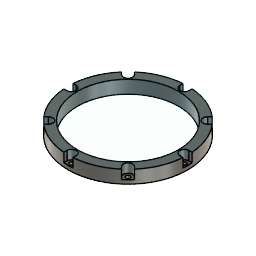
CycloidalDriveV1Assembly (Autodesk Fusion 360 archive; units mm, degrees)
design "CoperchioOutput2.0"
part number: 2026-04-16-14-40-12-138
Autodesk Fusion 360 part; units mm, degrees
sketch "Sketch1" plane through (0, 0, 0) normal (0, 0, 1) x (1, 0, 0)
  circle A0 centre (0, 0) radius 46
  circle A1 centre (0, 0) radius 38.925
  dimension "d1" = 92
  dimension "d2" = 77.85
  constraint coincident A0.centre A1.centre
  constraint concentric A0 A1
  measures "d1" diameter of A0
  measures "d2" diameter of A1
extrude "Extrude1" add sketch "Sketch1" along normal blind 10
sketch "Sketch2" plane through (0, 0, 10) normal (0, 0, 1) x (-1, 0, 0)
  circle A0 centre (0, 0) radius 38.925
  circle A1 centre (0, 0) radius 46
  circle A2 centre (0, -43.375) radius 1.65
  dimension "d5" = 3.3
  dimension "d6" = 43.375
  measures "d5" diameter of A2
  measures "d6" distance of A0.centre A2.centre
extrude "Extrude2" cut sketch "Sketch2" against normal blind 10 contours A2
sketch "Sketch3" plane through (0, 0, 10) normal (0, 0, 1) x (-1, 0, 0)
  circle A0 centre (0, -43.375) radius 1.65
  circle A1 centre (0, 0) radius 38.925
  circle A2 centre (0, 0) radius 46
pattern_circular "C-Pattern1" count 8 over 360 about axis through (0, 0, 1.75) along (0, 0, 1) of "Extrude2"
sketch "Sketch4" plane through (0, 0, 10) normal (0, 0, 1) x (-1, 0, 0)
  circle A0 centre (0, -43.375) radius 1.65
  line L0 (3.5, -43.375) -> (3.5, -46)
  line L1 (-3.5, -43.375) -> (-3.5, -46)
  arc A1 (3.5, -43.375) -> (-3.5, -43.375) centre (0, -43.375) ccw
  circle A2 centre (0, 0) radius 46
  dimension "d11" = 7
  constraint concentric A0 A1
  constraint tangent L0 A1
  constraint vertical L0
  constraint tangent L1 A1
  constraint vertical L1
  measures "d11" diameter of A1
extrude "Extrude3" cut sketch "Sketch4" against normal blind 7 contours L0 L1 A1 A2 picked at (-2.8289, -44.4442)
pattern_circular "C-Pattern2" count 8 over 360 about axis through (0, 0, 1.75) along (0, 0, 1) of "Extrude3"

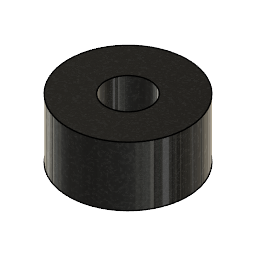
design "Cuscinetto 3x8x4"
part number: 2026-04-13-20-27-40-353
Autodesk Fusion 360 part; units mm, degrees
sketch "Sketch1" plane through (0, 0, 0) normal (0, 0, 1) x (1, 0, 0)
  circle A0 centre (0, 0) radius 1.5
  circle A1 centre (0, 0) radius 4
  dimension "d1" = 3
  dimension "d2" = 8
  constraint coincident A0.centre A1.centre
  constraint concentric A0 A1
  measures "d1" diameter of A0
  measures "d2" diameter of A1
extrude "Extrude1" add sketch "Sketch1" along normal blind 4

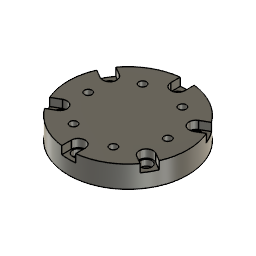
design "Output8mm2.0"
part number: 2026-04-23-17-57-34-450
Autodesk Fusion 360 part; units mm, degrees
sketch "Sketch1" plane through (0, 0, 0) normal (0, 0, 1) x (1, 0, 0)
  circle A0 centre (0, 0) radius 30
  dimension "d1" = 60
  constraint coincident A0.centre origin
  measures "d1" diameter of A0
extrude "Extrude1" add sketch "Sketch1" along normal blind 7
sketch "Sketch2" plane through (0, 0, 7) normal (0, 0, 1) x (-1, 0, 0)
  circle A0 centre (0, 0) radius 30
  line L0 (0, 0) -> (0, -25) construction
  circle A1 centre (0, -25) radius 2.825
  dimension "d4" = 5.65
  constraint coincident A0.centre L0.start
  constraint vertical L0
  constraint coincident L0.end A1.centre
  measures "d4" diameter of A1
extrude "Extrude2" cut sketch "Sketch2" against normal blind 3 contours A1
sketch "Sketch3" plane through (0, 0, 4) normal (0, 0, 1) x (-1, 0, 0)
  circle A0 centre (0, -25) radius 2.825
  circle A1 centre (0, -25) radius 1.675
  dimension "d7" = 3.35
  constraint concentric A0 A1
  measures "d7" diameter of A1
extrude "Extrude3" cut sketch "Sketch3" against normal blind 4 contours A1
pattern_circular "C-Pattern1" count 6 over 360 about axis through (0, 0, 1.75) along (0, 0, 1) of "Extrude2", "Extrude3"
sketch "Sketch5" plane through (0, 0, 7) normal (0, 0, 1) x (-1, 0, 0)
  circle A0 centre (0, 0) radius 30
  circle A1 centre (0, -25) radius 2.825
  circle A2 centre (21.6506, -12.5) radius 2.825
  circle A3 centre (21.6506, 12.5) radius 2.825
  circle A4 centre (0, 25) radius 2.825
  circle A5 centre (-21.6506, 12.5) radius 2.825
  circle A6 centre (-21.6506, -12.5) radius 2.825
  line L0 (-3.5, 25) -> (-3.5, 29.7951)
  line L1 (3.5, 25) -> (3.5, 29.7951)
  line L2 (0, 25) -> (0, 30) construction
  arc A7 (-3.5, 25) -> (3.5, 25) centre (0, 25) ccw
  circle A8 centre (0, 0) radius 30
  line L3 (-23.4006, 9.4689) -> (-27.5533, 11.8665)
  arc A9 (-23.4006, 9.4689) -> (-19.9006, 15.5311) centre (-21.6506, 12.5) ccw
  line L4 (-19.9006, 15.5311) -> (-24.0533, 17.9287)
  line L5 (-19.9006, -15.5311) -> (-24.0533, -17.9287)
  arc A10 (-19.9006, -15.5311) -> (-23.4006, -9.4689) centre (-21.6506, -12.5) ccw
  line L6 (-23.4006, -9.4689) -> (-27.5533, -11.8665)
  line L7 (3.5, -25) -> (3.5, -29.7951)
  arc A11 (3.5, -25) -> (-3.5, -25) centre (0, -25) ccw
  line L8 (-3.5, -25) -> (-3.5, -29.7951)
  line L9 (23.4006, -9.4689) -> (27.5533, -11.8665)
  arc A12 (23.4006, -9.4689) -> (19.9006, -15.5311) centre (21.6506, -12.5) ccw
  line L10 (19.9006, -15.5311) -> (24.0533, -17.9287)
  line L11 (19.9006, 15.5311) -> (24.0533, 17.9287)
  arc A13 (19.9006, 15.5311) -> (23.4006, 9.4689) centre (21.6506, 12.5) ccw
  line L12 (23.4006, 9.4689) -> (27.5533, 11.8665)
  dimension "d16" = 7
  dimension "d18" = 360
  constraint concentric A4 A7
  constraint coincident A0 L0.end
  constraint vertical L0
  constraint tangent L0 A7
  constraint coincident A0 L1.end
  constraint tangent L1 A7
  constraint coincident A4.centre L2.start
  constraint coincident A0 L2.end
  constraint vertical L2
  measures "d16" diameter of A7
extrude "Extrude5" add sketch "Sketch5" along normal blind 4 contours A0 L0 L1 A7 A8 L3 A9 L4 L5 A10 L6 L7 A11 L8 L9 A12 L10 L11 A13 L12
sketch "Sketch6" plane through (0, 0, 11) normal (0, 0, 1) x (-1, 0, 0)
  line L0 (19.9006, 15.5311) -> (24.0533, 17.9287)
  arc A0 (24.0533, 17.9287) -> (3.5, 29.7951) centre (0, 0) ccw
  line L1 (3.5, 29.7951) -> (3.5, 25)
  arc A1 (-3.5, 25) -> (3.5, 25) centre (0, 25) ccw
  line L2 (-3.5, 25) -> (-3.5, 29.7951)
  arc A2 (-3.5, 29.7951) -> (-24.0533, 17.9287) centre (0, 0) ccw
  line L3 (-24.0533, 17.9287) -> (-19.9006, 15.5311)
  arc A3 (-23.4006, 9.4689) -> (-19.9006, 15.5311) centre (-21.6506, 12.5) ccw
  line L4 (-23.4006, 9.4689) -> (-27.5533, 11.8665)
  arc A4 (-27.5533, 11.8665) -> (-27.5533, -11.8665) centre (0, 0) ccw
  line L5 (-27.5533, -11.8665) -> (-23.4006, -9.4689)
  arc A5 (-19.9006, -15.5311) -> (-23.4006, -9.4689) centre (-21.6506, -12.5) ccw
  line L6 (-19.9006, -15.5311) -> (-24.0533, -17.9287)
  arc A6 (-24.0533, -17.9287) -> (-3.5, -29.7951) centre (0, 0) ccw
  line L7 (-3.5, -29.7951) -> (-3.5, -25)
  arc A7 (3.5, -25) -> (-3.5, -25) centre (0, -25) ccw
  line L8 (3.5, -25) -> (3.5, -29.7951)
  arc A8 (3.5, -29.7951) -> (24.0533, -17.9287) centre (0, 0) ccw
  line L9 (24.0533, -17.9287) -> (19.9006, -15.5311)
  arc A9 (23.4006, -9.4689) -> (19.9006, -15.5311) centre (21.6506, -12.5) ccw
  line L10 (23.4006, -9.4689) -> (27.5533, -11.8665)
  arc A10 (27.5533, -11.8665) -> (27.5533, 11.8665) centre (0, 0) ccw
  line L11 (27.5533, 11.8665) -> (23.4006, 9.4689)
  arc A11 (19.9006, 15.5311) -> (23.4006, 9.4689) centre (21.6506, 12.5) ccw
  circle A12 centre (-20, 0) radius 1.9
  line L12 (-20, 0) -> (0, 0) construction
  dimension "d21" = 3.8
  constraint coincident A12.centre L12.start
  constraint coincident A0.centre A2.centre
  constraint horizontal L12
  measures "d21" diameter of A12
extrude "Extrude6" cut sketch "Sketch6" against normal blind 5.2 contours A12
pattern_circular "C-Pattern2" count 6 over 360 about axis through (0, 0, 1.75) along (0, 0, 1) of "Extrude6"

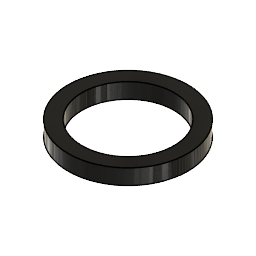
design "Cuscinetto 60x78x10"
part number: 2026-04-15-21-13-08-040
Autodesk Fusion 360 part; units mm, degrees
sketch "Sketch1" plane through (0, 0, 0) normal (0, 0, 1) x (1, 0, 0)
  circle A0 centre (0, 0) radius 30
  circle A1 centre (0, 0) radius 39
  dimension "d1" = 60
  dimension "d2" = 78
  constraint coincident A0.centre A1.centre
  constraint concentric A0 A1
  measures "d1" diameter of A0
  measures "d2" diameter of A1
extrude "Extrude1" add sketch "Sketch1" along normal blind 10

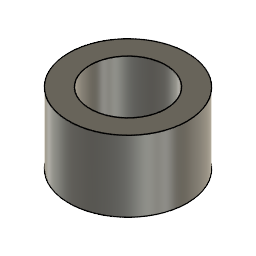
design "Spaziatore2"
part number: 2026-04-16-14-43-29-864
Autodesk Fusion 360 part; units mm, degrees
sketch "Sketch1" plane through (0, 0, 0) normal (0, 0, 1) x (1, 0, 0)
  circle A0 centre (0, 0) radius 2.5
  circle A1 centre (0, 0) radius 1.6
  dimension "d1" = 5
  dimension "d2" = 3.2
  constraint coincident A0.centre A1.centre
  constraint concentric A0 A1
  measures "d1" diameter of A0
  measures "d2" diameter of A1
extrude "Extrude1" add sketch "Sketch1" along normal blind 3

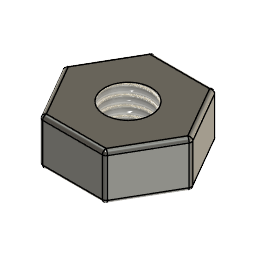
design "M3Bolt"
part number: 2026-08-22-12-33-28-107
Autodesk Fusion 360 part; units mm, degrees
sketch "Sketch1" plane through (0, 0, 0) normal (0, 0, 1) x (1, 0, 0)
  line L0 (-1.7321, 3) -> (-3.4641, 0)
  line L1 (-3.4641, 0) -> (-1.7321, -3)
  line L2 (-1.7321, -3) -> (1.7321, -3)
  line L3 (1.7321, -3) -> (3.4641, 0)
  line L4 (3.4641, 0) -> (1.7321, 3)
  line L5 (1.7321, 3) -> (-1.7321, 3)
  circle A0 centre (0, 0) radius 1.5
  dimension "d1" = 3
  dimension "d2" = 3
  constraint coincident A0.centre origin
  measures "d1" distance of A0.centre L5
  measures "d2" diameter of A0
extrude "Extrude1" add sketch "Sketch1" along normal blind 2.5
fillet "Fillet1" radius 0.2 18 edges at (2.5981, -1.5, 2.5) (0, -3, 2.5) (-2.5981, -1.5, 2.5) (-2.5981, 1.5, 2.5) (0, 3, 2.5) (1.7321, -3, 1.25) (3.4641, 0, 1.25) (2.5981, 1.5, 2.5) (1.7321, 3, 1.25) (-1.7321, 3, 1.25) (2.5981, 1.5, 0) (0, 3, 0) (-3.4641, 0, 1.25) (-2.5981, 1.5, 0) (-2.5981, -1.5, 0) (-1.7321, -3, 1.25) (0, -3, 0) (2.5981, -1.5, 0)
thread "Thread1" "ISO Metric profile 3.0 M3x0.5 M3x0.5 6H" major diameter 3.086 minor diameter 2.529 pitch 0.5 angle 60 resizes the face on face at (1.4981, -0.0748, 1.6667)

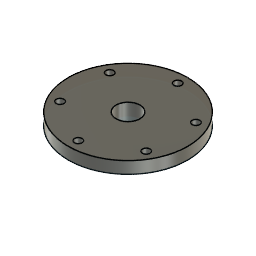
design "OutPutShaft2.0"
part number: 2026-04-23-18-12-03-313
Autodesk Fusion 360 part; units mm, degrees
sketch "Sketch1" plane through (0, 0, 0) normal (0, 0, 1) x (1, 0, 0)
  circle A0 centre (0, 0) radius 30
  dimension "d1" = 60
  constraint coincident A0.centre origin
  measures "d1" diameter of A0
extrude "Extrude1" add sketch "Sketch1" along normal blind 6
sketch "Sketch2" plane through (0, 0, 6) normal (0, 0, 1) x (-1, 0, 0)
  circle A0 centre (0, 0) radius 30
  line L0 (0, 0) -> (0, -25) construction
  circle A1 centre (0, -25) radius 1.9
  dimension "d4" = 25
  dimension "d5" = 3.8
  constraint coincident A0.centre L0.start
  constraint vertical L0
  constraint coincident L0.end A1.centre
  measures "d4" distance of A0.centre L0.end
  measures "d5" diameter of A1
extrude "Extrude2" cut sketch "Sketch2" against normal blind 5.2 contours A1
sketch "Sketch3" plane through (0, 0, 0) normal (0, 0, -1) x (1, 0, 0)
  circle A0 centre (0, 0) radius 30
pattern_circular "C-Pattern1" count 6 over 360 about axis through (0, 0, 1.75) along (0, 0, 1) of "Extrude2"
sketch "Sketch4" plane through (0, 0, 0) normal (0, 0, -1) x (1, 0, 0)
  circle A0 centre (0, 0) radius 10.05
  dimension "d10" = 20.1
  constraint coincident A0.centre origin
  measures "d10" diameter of A0
extrude "Extrude3" add sketch "Sketch4" along normal blind 8
sketch "Sketch5" plane through (0, 0, -8) normal (0, 0, -1) x (1, 0, 0)
  circle A0 centre (0, 0) radius 10.05
  circle A1 centre (0, 0) radius 6
  dimension "d13" = 12
  constraint concentric A0 A1
  measures "d13" diameter of A1
extrude "Extrude4" cut sketch "Sketch5" against normal blind 14 contours A1

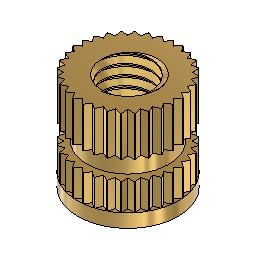
design "_brass+insert+M3.cf30406c-077e-4d83-afc2-e8e3747f2743"
Autodesk Fusion 360 part; units mm, degrees
sketch "Sketch1" plane through (0, 0, 0) normal (1, 0, 0) x (0, 1, 0)
  line L0 (0, 0) -> (-2.625, 0)
  line L1 (-2.625, 0) -> (-2.625, 2.1)
  line L2 (-2.625, 2.1) -> (-2.125, 2.1)
  line L3 (-2.125, 2.1) -> (-2.125, 3.1)
  line L4 (-2.125, 3.1) -> (-2.625, 3.1)
  line L5 (-2.625, 3.1) -> (-2.625, 5.2)
  line L6 (-2.625, 5.2) -> (0, 5.2)
  line L7 (0, 5.2) -> (0, 0)
  dimension "d1" = 5.2
  dimension "d2" = 2.625
  dimension "d3" = 1
  dimension "d4" = 0.5
  measures "d1" distance of L0.start
revolve "Revolve1" add sketch "Sketch1" angle 360 about axis through (0, 0, 5.2) along (0, 0, -1)
hole "Hole1" at (0, 0, 5.2) direction (0, 0, -1) diameter 2.529 depth 2.5 tip angle 118
thread "Thread1" "ISO Metric profile 3.0 M3x0.5 6H" major diameter 3.086 minor diameter 2.529 pitch 0.5 angle 60 modelled right hand crest width 0.0625 on face at (0.063, -1.2629, 4.3667) crest through (1.2645, 0, 5.4812)
sketch "Sketch2" plane through (0, 0, 5.2) normal (0, 0, 1) x (-1, 0, 0)
  circle A0 centre (0, 0) radius 2.625
  line L0 (0.2391, -2.6141) -> (0, -2.375)
  line L1 (0, -2.375) -> (-0.2391, -2.6141)
  line L2 (0, -2.375) -> (0, -2.625) construction
  dimension "d9" = 90
  dimension "d10" = 0.25
  measures "d9" angle of L0 L1
extrude "Extrude1" cut sketch "Sketch2" against normal blind 4.5 contours A0 L0 L1 picked at (0, -2.5409)
pattern_circular "C-Pattern1" count 32 over 360 about axis through (0, 0, 1.75) along (0, 0, 1) of "Extrude1"
equation "d2 = 5.25 mm / 2"

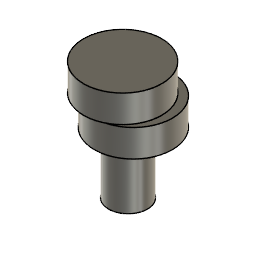
design "AlberoCicloide3"
part number: 2026-04-16-15-20-54-284
Autodesk Fusion 360 part; units mm, degrees
sketch "Sketch1" plane through (0, 0, 0) normal (0, 0, 1) x (1, 0, 0)
  circle A0 centre (0, 0) radius 5
  dimension "d1" = 10
  constraint coincident A0.centre origin
  measures "d1" diameter of A0
extrude "Extrude1" add sketch "Sketch1" along normal blind 18
ref_plane "WorkPlane1" through (0, 0, 17) normal (0, 0, 1) x (1, 0, 0)
ref_plane "WorkPlane2" through (0, 0, 1) normal (0, 0, -1) x (-1, 0, 0)
sketch "Sketch2" plane through (0, 0, 17) normal (0, 0, 1) x (1, 0, 0)
  line L0 (0, 0) -> (0, -1.37) construction
  circle A0 centre (0, -1.37) radius 9.925
  dimension "d15" = 1.37
  dimension "d16" = 19.85
  constraint coincident L0.start origin
  constraint vertical L0
  constraint coincident L0.end A0.centre
  measures "d15" distance of L0.start L0.end
  measures "d16" diameter of A0
extrude "Extrude2" add sketch "Sketch2" against normal blind 7
sketch "Sketch3" plane through (0, 0, 1) normal (0, 0, -1) x (-1, 0, 0)
  line L0 (0, 0) -> (0, 1.37) construction
  circle A0 centre (0, 1.37) radius 9.925
  dimension "d17" = 1.37
  dimension "d18" = 19.85
  constraint coincident L0.start origin
  constraint vertical L0
  constraint coincident L0.end A0.centre
  measures "d17" distance of L0.start L0.end
  measures "d18" diameter of A0
extrude "Extrude3" add sketch "Sketch3" against normal blind 7
sketch "Sketch4" plane through (0, 0, 0) normal (0, 0, -1) x (1, 0, 0)
  circle A0 centre (0, 0) radius 5
  arc A1 (1.59, -2.12) -> (-1.59, -2.12) centre (0, 0) ccw
  line L0 (-1.59, -2.12) -> (1.59, -2.12)
extrude "Extrude4" cut sketch "Sketch4" against normal blind 15 contours A1 L0
extrude "Extrude5" add 1 faces at (0.1246, 3.0753, 0) along direction (0, 0, -1) blind 14
extrude "Extrude6" cut 1 faces at (1.3101, -1.9935, 18) along direction (0, 0, -1) blind 1
sketch "Sketch5" plane through (0, 0, 17) normal (0, 0, 1) x (-1, 0, 0)
  circle A0 centre (0, 1.37) radius 9.925
  circle A1 centre (0, 1.37) radius 10.005
  dimension "d21" = 0.08
extrude "Extrude7" add sketch "Sketch5" against normal blind 7
sketch "Sketch6" plane through (0, 0, 8) normal (0, 0, 1) x (-1, 0, 0)
  circle A0 centre (0, -1.37) radius 9.925
  circle A1 centre (0, 0) radius 5
  circle A2 centre (0, -1.37) radius 10.005
  dimension "d24" = 0.08
extrude "Extrude8" add sketch "Sketch6" against normal blind 7 contours A2

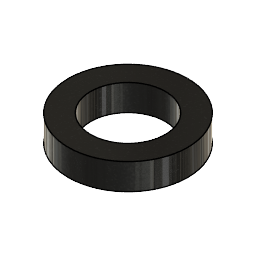
design "Cuscinetto 20x32x7"
part number: 2026-04-13-20-22-04-809
Autodesk Fusion 360 part; units mm, degrees
sketch "Sketch1" plane through (0, 0, 0) normal (0, 0, 1) x (1, 0, 0)
  circle A0 centre (0, 0) radius 10
  circle A1 centre (0, 0) radius 16
  dimension "d1" = 20
  dimension "d2" = 32
  constraint coincident A0.centre A1.centre
  constraint concentric A0 A1
  measures "d1" diameter of A0
  measures "d2" diameter of A1
extrude "Extrude1" add sketch "Sketch1" along normal blind 7

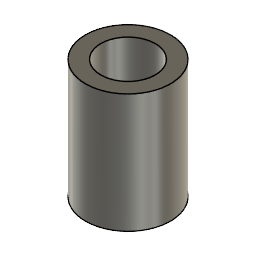
design "Spaziatore1"
part number: 2026-04-16-14-43-29-864
Autodesk Fusion 360 part; units mm, degrees
sketch "Sketch1" plane through (0, 0, 0) normal (0, 0, 1) x (1, 0, 0)
  circle A0 centre (0, 0) radius 2.5
  circle A1 centre (0, 0) radius 1.6
  dimension "d1" = 5
  dimension "d2" = 3.2
  constraint coincident A0.centre A1.centre
  constraint concentric A0 A1
  measures "d1" diameter of A0
  measures "d2" diameter of A1
extrude "Extrude1" add sketch "Sketch1" along normal blind 7
